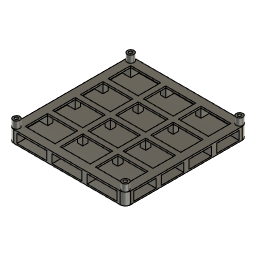
board_holder_no_ziptie (Autodesk Fusion 360 design; units mm, degrees)
Autodesk Fusion 360 part; units mm, degrees
sketch "Sketch1" plane through (0, 0, 0) normal (0, 0, 1) x (1, 0, 0)
  line L0 (-62, -65) -> (62, -65) construction
  line L1 (62, -65) -> (62, 65) construction
  line L2 (62, 65) -> (-62, 65) construction
  line L3 (-62, 65) -> (-62, -65) construction
  line L4 (-62, -65) -> (62, 65) construction
  line L5 (62, -65) -> (-62, 65) construction
  circle A0 centre (-62, 65) radius 1.85
  circle A1 centre (62, 65) radius 1.85
  circle A2 centre (-62, -65) radius 1.85
  circle A3 centre (62, -65) radius 1.85
  line L6 (-66.5, 69.5) -> (66.5, 69.5)
  line L7 (66.5, 69.5) -> (66.5, -69.5)
  line L8 (66.5, -69.5) -> (-66.5, -69.5)
  line L9 (-66.5, -69.5) -> (-66.5, 69.5)
  line L10 (-66.5, 69.5) -> (66.5, -69.5) construction
  line L11 (66.5, 69.5) -> (-66.5, -69.5) construction
  circle A4 centre (-62, 65) radius 3.85
  circle A5 centre (62, 65) radius 3.85
  circle A6 centre (-62, -65) radius 3.85
  circle A7 centre (62, -65) radius 3.85
  dimension "d1" = 124
  dimension "d2" = 130
  dimension "d3" = 3.7
  dimension "d6" = 124
  dimension "d8" = 133
  dimension "d9" = 7.7
  dimension "d12" = 124
  dimension "d102" = 139
  constraint perpendicular L0 L1
  constraint parallel L0 L2
  constraint parallel L1 L3
  constraint horizontal L0
  constraint coincident L4 origin
  constraint coincident L5 origin
  constraint coincident L2.end L3.start
  constraint perpendicular L6 L7
  constraint parallel L6 L8
  constraint parallel L7 L9
  constraint horizontal L6
  constraint coincident L10 origin
  constraint coincident L11 origin
  constraint concentric A0 A4
  measures "d1" distance of L1.end L2.end
  measures "d2" distance of L0.end L1.end
  measures "d3" diameter of A0
  measures "d8" distance of L7.end L8.end
  measures "d9" diameter of A4
  measures "d102" distance of L6.start L8.end L0.start
extrude "Extrude1" add sketch "Sketch1" along normal blind 20 contours A4 | A5 | A6 | A7 makes body 1 at (-64.2474, 68.126, 13.3333) makes body 2 at (65.3812, 66.8413, 6.6667) makes body 3 at (-58.1548, -64.8081, 6.6667) makes body 4 at (58.3822, -66.3168, 13.3333)
extrude "Extrude2" add sketch "Sketch1" against normal blind 2 contours L6 L7 L8 L9 | A4 | A5 | A6 | A7 bodies 1 2 3 4
extrude "Extrude3" add sketch "Sketch1" along normal blind 12 contours L6 L7 L8 L9 bodies 1
sketch "Sketch2" plane through (0, -69.5, 0) normal (0, -1, 0) x (1, 0, 0)
  line L0 (66.5, -2) -> (66.5, 12)
  line L1 (-66.5, 12) -> (-57, 12)
  line L2 (-57, 12) -> (-57, -2)
  line L3 (-57, -2) -> (-66.5, -2)
  line L4 (-66.5, -2) -> (-66.5, 12)
  line L5 (-57, 12) -> (-23, 12)
  line L6 (-23, 12) -> (-23, -2)
  line L7 (-23, -2) -> (-57, -2)
  line L8 (-57, -2) -> (-57, 12)
  line L9 (-66.5, 12) -> (-66.5, 10)
  line L10 (-66.5, -2) -> (-66.5, 0)
  line L11 (-66.5, 10) -> (66.5, 10)
  line L12 (-66.5, 0) -> (66.5, 0)
  point P0 (-66.5, 12)
  dimension "d64" = 14
  dimension "d65" = 9.5
  dimension "d66" = 14
  dimension "d67" = 34
  dimension "d68" = 2
  dimension "d69" = 2
  constraint horizontal L1
  constraint vertical L2
  constraint horizontal L3
  constraint vertical L4
  constraint horizontal L5
  constraint vertical L6
  constraint horizontal L7
  constraint vertical L8
  constraint perpendicular L1 L9
  constraint perpendicular L3 L10
  constraint coincident L0 L11.end
  constraint perpendicular L0 L11
  constraint coincident L0 L12.end
  constraint perpendicular L0 L12
  constraint coincident P0 L1.start
  measures "d64" distance of P0 L3.end
  measures "d65" distance of P0 L1.end
  measures "d66" distance of L1.end L2.end
  measures "d67" distance of L1.end L5.end
  measures "d68" distance of P0 L9.end
  measures "d69" distance of L3.end L10.end
sketch "Sketch3" plane through (66.5, 0, 0) normal (1, 0, 0) x (0, 1, 0)
  line L0 (-69.5, 12) -> (-69.5, -2)
  line L1 (-69.5, -2) -> (69.5, -2)
  line L2 (69.5, -2) -> (69.5, 12)
  line L3 (69.5, 12) -> (-69.5, 12)
  line L4 (-69.5, 12) -> (-60, 12)
  line L5 (-60, 12) -> (-60, -2)
  line L6 (-60, -2) -> (-69.5, -2)
  line L7 (-69.5, -2) -> (-69.5, 12)
  line L8 (-60, 12) -> (-34.5, 12)
  line L9 (-34.5, 12) -> (-34.5, -2)
  line L10 (-34.5, -2) -> (-60, -2)
  line L11 (-60, -2) -> (-60, 12)
  line L12 (-69.5, 12) -> (-69.5, 10)
  line L13 (-69.5, -2) -> (-69.5, 0)
  line L14 (-69.5, 10) -> (69.5, 10)
  line L15 (-69.5, 0) -> (69.5, 0)
  dimension "d85" = 9.5
  dimension "d86" = 14
  dimension "d87" = 25.5
  dimension "d88" = 14
  dimension "d89" = 2
  dimension "d90" = 2
  constraint horizontal L4
  constraint vertical L5
  constraint horizontal L6
  constraint vertical L7
  constraint coincident L0.start L3.end
  constraint horizontal L8
  constraint vertical L9
  constraint horizontal L10
  constraint vertical L11
  constraint perpendicular L3 L12
  constraint coincident L0.end L1.start
  constraint perpendicular L6 L13
  constraint coincident L2 L14.end
  constraint perpendicular L2 L14
  constraint coincident L2 L15.end
  constraint perpendicular L2 L15
  measures "d85" distance of L0.start L4.end
  measures "d86" distance of L0.start L0.end
  measures "d87" distance of L4.end L8.end
  measures "d88" distance of L4.end L5.end
  measures "d89" distance of L0.start L12.end
  measures "d90" distance of L0.end L13.end
sketch "Sketch4" plane through (0, 0, -2) normal (0, 0, -1) x (1, 0, 0)
  circle A0 centre (-62, 65) radius 1.85
  circle A1 centre (62, 65) radius 1.85
  line L0 (66.5, 69.5) -> (-66.5, 69.5)
  line L1 (-66.5, 69.5) -> (-66.5, -69.5)
  line L2 (-66.5, -69.5) -> (66.5, -69.5)
  line L3 (66.5, -69.5) -> (66.5, 69.5)
  line L4 (62, 65) -> (35, 65)
  line L5 (35, 65) -> (35, 38)
  line L6 (35, 38) -> (62, 38)
  line L7 (62, 38) -> (62, 65)
  circle A2 centre (35, 38) radius 6.5
  circle A3 centre (-62, -65) radius 1.85
  circle A4 centre (62, -65) radius 1.85
  dimension "d43" = 27
  dimension "d44" = 27
  dimension "d45" = 13
  constraint horizontal L4
  constraint vertical L5
  constraint horizontal L6
  constraint vertical L7
  constraint coincident A1.centre L4.start
  constraint coincident L5.end L6.start
  measures "d43" distance of A1.centre L4.end
  measures "d44" distance of A1.centre L6.end
  measures "d45" diameter of A2
extrude "Extrude10" cut sketch "Sketch3" against normal blind 133 contours L5 L9 L11 L14 L15 bodies 1
pattern_linear "R-Pattern2" count 4 spacing 31.5 along (0, 1, 0) of "Extrude10"
extrude "Extrude9" cut sketch "Sketch2" against normal blind 139 contours L2 L6 L8 L11 L12 bodies 1
pattern_linear "R-Pattern1" count 3 spacing 40 along (1, 0, 0) of "Extrude9"
ref_plane "WorkPlane1" through (0, 0, 12) normal (0, 0, 1) x (1, 0, 0)
sketch "Sketch6" plane through (0, 0, 12) normal (0, 0, 1) x (1, 0, 0)
  line L0 (-66.5, 69.5) -> (66.5, 69.5) construction
  line L1 (66.5, 69.5) -> (66.5, -69.5) construction
  line L2 (66.5, -69.5) -> (-66.5, -69.5) construction
  line L3 (-66.5, -69.5) -> (-66.5, 69.5) construction
  line L4 (-66.5, 69.5) -> (66.5, -69.5) construction
  line L5 (66.5, 69.5) -> (-66.5, -69.5) construction
  line L6 (-66.5, -69.5) -> (-57, -69.5) construction
  line L7 (-57, -69.5) -> (-57, -60) construction
  line L8 (-57, -60) -> (-66.5, -60) construction
  line L9 (-66.5, -60) -> (-66.5, -69.5) construction
  line L10 (-57, -60) -> (-23, -60)
  line L11 (-23, -60) -> (-23, -34.5)
  line L12 (-23, -34.5) -> (-57, -34.5)
  line L13 (-57, -34.5) -> (-57, -60)
  dimension "d106" = 133
  dimension "d107" = 139
  dimension "d108" = 9.5
  dimension "d109" = 9.5
  dimension "d110" = 34
  dimension "d111" = 25.5
  constraint perpendicular L0 L1
  constraint parallel L0 L2
  constraint parallel L1 L3
  constraint horizontal L0
  constraint coincident L4 origin
  constraint coincident L5 origin
  constraint horizontal L6
  constraint vertical L7
  constraint horizontal L8
  constraint vertical L9
  constraint horizontal L10
  constraint vertical L11
  constraint horizontal L12
  constraint vertical L13
  measures "d106" distance of L1.end L2.end
  measures "d107" distance of L0.end L1.end
  measures "d108" distance of L2.end L6.end
  measures "d109" distance of L2.end L8.end
  measures "d110" distance of L7.end L10.end
  measures "d111" distance of L7.end L12.end
extrude "Extrude11" cut sketch "Sketch6" against normal blind 2 bodies 1
pattern_linear "R-Pattern3" count 4 spacing 31.5 along (0, 1, 0) count 3 spacing 40 along (1, 0, 0) of "Extrude11"
fillet "Fillet1" radius 6 4 edges at (-66.5, -69.5, 5) (66.5, -69.5, 5) (66.5, 69.5, 5) (-66.5, 69.5, 5) on bodies 1
chamfer "Chamfer3" distance 0.4 angle 45 12 edges at (-63.7248, -65.669, -2) (60.2752, -65.669, -2) (60.2752, 64.331, -2) (-63.7248, 64.331, -2) (0, 69.5, -2) (-64.7426, 67.7426, -2) (-66.5, 0, -2) (-64.7426, -67.7426, -2) (0, -69.5, -2) (64.7426, -67.7426, -2) (66.5, 0, -2) (64.7426, 67.7426, -2) on bodies 1
equation "d1 = PWidth"
equation "d2 = PLength"
equation "d6 = PWidth"
equation "d7 = -PLength"
equation "d8 = BWidth"
equation "d9 = d3 + 4 mm"
equation "d12 = PWidth"
equation "d13 = -PLength"
equation "d14 = PegH"
equation "d16 = -Bottom"
equation "d18 = InnerHeight + Top"
equation "BWidth = PWidth + 9 mm"
equation "Ends = 9.5 mm"
equation "InnerWalls = 6 mm"
equation "InnerHeight = 10 mm"
equation "XChamberW = ( ( BWidth - ( Ends * 2 ) - ( InnerWalls * ( XChannels - 1 ) ) ) / XChannels )"
equation "Bottom = 2 mm"
equation "Top = 2 mm"
equation "XChamberH = Bottom + Top + InnerHeight"
equation "PegH = 22 mm - Bottom"
equation "d64 = XChamberH"
equation "d65 = Ends"
equation "d66 = XChamberH"
equation "d67 = XChamberW"
equation "d68 = Top"
equation "d69 = Bottom"
equation "XChannels = 3"
equation "d79 = -BLength"
equation "d81 = XChannels"
equation "d83 = -( XChamberW + InnerWalls ) * ( XChannels - 1 )"
equation "d85 = Ends"
equation "d86 = XChamberH"
equation "d87 = YChamberW"
equation "d88 = YChamberH"
equation "d89 = Top"
equation "d90 = Bottom"
equation "d91 = -BWidth"
equation "d93 = YChannels"
equation "d95 = ( YChamberW + InnerWalls ) * ( YChannels - 1 )"
equation "BLength = PLength + 9 mm"
equation "YChamberW = ( ( BLength - ( Ends * 2 ) - ( InnerWalls * ( YChannels - 1 ) ) ) / YChannels )"
equation "YChamberH = Bottom + Top + InnerHeight"
equation "YChannels = 4"
equation "d102 = BLength"
equation "PWidth = 124 mm"
equation "PLength = 130 mm"
equation "d105 = InnerHeight + Top"
equation "d106 = BWidth"
equation "d107 = BLength"
equation "d108 = Ends"
equation "d109 = Ends"
equation "d110 = XChamberW"
equation "d111 = YChamberW"
equation "d112 = -Top"
equation "d114 = YChannels"
equation "d115 = XChannels"
equation "d116 = ( YChamberW + InnerWalls ) * ( YChannels - 1 )"
equation "d117 = -( XChamberW + InnerWalls ) * ( XChannels - 1 )"
